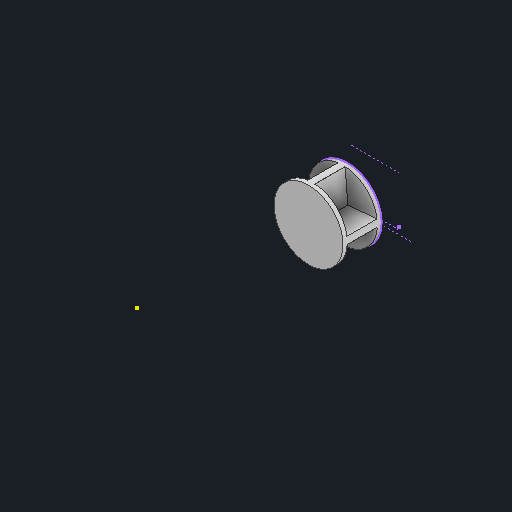
# Autodesk Inventor part: wheel
Saved by Autodesk Inventor 2026.2 (Build 302298000, 298)
## iProperties
Created: 2026-03-14
Part Number: wheel
Material: Generic
Document SubType Name: Modeling
Designer: danda
Density: 1 g/cm^3
Appearance: Default
Author: danda
Autodesk Inventor part; units mm, degrees
ref_plane "YZ Plane" through (0, 0, 0) normal (1, 0, 0) x (0, 1, 0)
ref_plane "XZ Plane" through (0, 0, 0) normal (0, 1, 0) x (-1, 0, 0)
ref_plane "XY Plane" through (0, 0, 0) normal (0, 0, 1) x (1, 0, 0)
sketch "Sketch1" plane through (0, 0, 0) normal (0, 0, 1) x (1, 0, 0)
  line L0 (204.17, 231.1255) -> (241.5918, 231.1255)
  line L1 (241.5918, 231.1255) -> (284.0136, 231.1255)
  line L2 (204.17, 226.1255) -> (241.5918, 226.1255)
  line L3 (246.5918, 226.1255) -> (284.0136, 226.1255)
  line L4 (246.5918, 188.7037) -> (246.5918, 226.1255)
  line L5 (246.5918, 231.1255) -> (246.5918, 268.5473)
  line L6 (241.5918, 188.7037) -> (241.5918, 226.1255)
  line L7 (241.5918, 231.1255) -> (241.5918, 268.5473)
  line L8 (241.5918, 231.1255) -> (288.8318, 231.1255) construction
  line L9 (246.5918, 231.1255) -> (303.9178, 231.1255) construction
  line L10 (246.5918, 288.5734) -> (304.1186, 288.5734) construction
  circle A0 centre (244.0918, 228.6255) radius 40
  line L11 (246.5918, 226.1255) -> (249.8364, 189.0401)
  line L12 (246.5918, 226.1255) -> (283.8188, 226.1255) construction
  line L13 (283.8188, 226.1255) -> (246.5918, 222.8685)
  line L14 (283.8188, 226.1255) -> (321.1881, 226.1255) construction
  line L15 (246.5918, 231.1255) -> (283.6772, 234.37)
  line L16 (246.5918, 268.3525) -> (249.8488, 231.1255)
  line L17 (241.5918, 231.1255) -> (238.3473, 268.2108)
  line L18 (204.3648, 231.1255) -> (241.5918, 234.3824)
  line L19 (241.5918, 226.1255) -> (204.5065, 222.8809)
  line L20 (241.5918, 188.8985) -> (238.3349, 226.1255)
  point P0 (0, 0)
  point P1 (303.8392, 234.1257)
  point P2 (241.3091, 234.3577)
  point P3 (249.824, 231.4082)
  point P4 (238.3596, 225.8427)
  point P5 (246.8746, 222.8933)
  dimension "d31" = 80
  dimension "d33" = 85
  dimension "d34" = 175
  dimension "d37" = 360
  constraints: 42 end point, 8 parallel, 5 horizontal, 2 equal length, 2 point on line, 36 other
  measures "d33" angle of L11 L12
  measures "d34" angle of L13 L14
extrude "Extrusion1" add sketch "Sketch1" along normal blind 45
extrude "Extrusion2" cut sketch "Sketch1" along normal blind 40 contours A0 L17 L18 L0 | L19 L20 L6 A0 | A0 L15 L16 L5 | L11 L13 L3 A0
extrude "Extrusion4" add sketch "Sketch1" along normal blind 5 contours A0 L17 L18 L0 | L19 L20 L6 A0 | A0 L15 L16 L5 | L11 L13 L3 A0
ref_plane "Work Plane1" through (244.0918, 228.6255, 0) normal (0, 0, -1) x (-1, 0, 0)
sketch "Sketch2" plane through (244.0918, 228.6255, 0) normal (0, 0, -1) x (-1, 0, 0)
  circle A0 centre (0, 0) radius 4
  point P0 (244.0918, -228.6255)
  dimension "d28" = 8
  constraints: 1 centre point
  measures "d28" diameter of A0
extrude "Extrusion5" cut sketch "Sketch2" against normal blind 10
body "Solid1"
